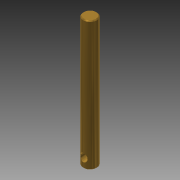
# Autodesk Inventor part: Link Arm1
Saved by Autodesk Inventor 2013 (Build 170138000, 138)
## iProperties
Created: 2012-10-29
Part Number: Link Arm1
Material: Generic
Document SubType Name: Modeling
Designer: uqgtayle
Density: 1 g/cm^3
Author: uqgtayle
Autodesk Inventor part; units mm, degrees
ref_plane "YZ Plane" through (0, 0, 0) normal (1, 0, 0) x (0, 1, 0)
ref_plane "XZ Plane" through (0, 0, 0) normal (0, 1, 0) x (-1, 0, 0)
ref_plane "XY Plane" through (0, 0, 0) normal (0, 0, 1) x (1, 0, 0)
sketch "Sketch1" plane through (0, 0, 0) normal (0, 0, 1) x (1, 0, 0)
  circle A0 centre (0, 0) radius 2
  dimension "d0" = 4
  constraints: 1 centre point, 1 coincident
  measures "d0" diameter of A0
extrude "Extrusion1" add sketch "Sketch1" along normal blind 38
ref_plane "Work Plane1" through (6.4921, 0, 2.8) normal (0, -0.9961947, -0.0871557) x (-1, 0, 0)
sketch "Sketch3" plane through (6.4921, 0, 2.8) normal (0, -0.9961947, -0.0871557) x (-1, 0, 0)
  ellipse E0 centre (6.4921, 0) end of major axis (6.4921, -22.9474) minor radius 2 (4.5072, 2.8107) -> (8.477, 2.8107) ccw projected
  line L0 (4.5072, 2.8107) -> (8.477, 2.8107) projected
  ellipse E1 centre (6.4921, 2.7893) end of major axis (8.4921, 2.7893) minor radius 0.1743 projected
  circle A0 centre (6.4921, 0) radius 1
  point P0 (6.4921, -0.0107)
  dimension "d6" = 2.8
  dimension "d14" = 2
  constraints: 1 centre point, 1 coincident, 2 other
  measures "d6" distance of point (6.492, -0.011) point (6.492, 2.789)
  measures "d14" diameter of A0
extrude "Extrusion2" cut sketch "Sketch3" along normal through all both and the other way through all contours A0
ref_plane "Work Plane2" through (6.4921, 0, 2.8) normal (0, -0.9961947, 0.0871557) x (-1, 0, 0)
sketch "Sketch5" plane through (6.4921, 0, 2.8) normal (0, -0.9961947, 0.0871557) x (-1, 0, 0)
  circle A0 centre (6.4921, 0.0156) radius 1
  point P0 (6.4921, 2.7893)
  dimension "d18" = 2
  constraints: 1 centre point
  measures "d18" diameter of A0
extrude "Extrusion3" cut sketch "Sketch5" along normal through all both and the other way through all
chamfer "Chamfer1" distance 0.25 angle 45 2 edges at (-2, 0, 38) (-2, 0, 0)
body "Solid1"
